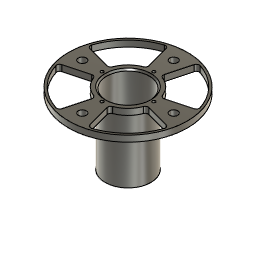
Top fan tube (Autodesk Fusion 360 design; units mm, degrees)
Autodesk Fusion 360 part; units mm, degrees
sketch "Sketch1" plane through (0, 0, 0) normal (0, 0, 1) x (1, 0, 0)
  circle A0 centre (0, 0) radius 39
  circle A1 centre (0, 0) radius 14
  circle A2 centre (0, 0) radius 17 construction
  circle A3 centre (0, 0) radius 17.5
  circle A4 centre (0, 0) radius 37.5
  line L0 (0, 0) -> (-11.368, 42.4258)
  line L1 (0, 0) -> (43.9224, 0) construction
  line L2 (0, 0) -> (10.4937, -39.163)
  line L3 (0, 0) -> (40.5446, 0) construction
  line L4 (0, 0) -> (-10.0939, -37.6711)
  line L5 (0, 0) -> (39, 0) construction
  line L6 (0, 0) -> (15.1457, 56.5247)
  line L7 (0, 0) -> (58.5186, 0) construction
  line L8 (0, 0) -> (-54.6126, 14.6334)
  line L9 (0, 0) -> (56.5391, 0) construction
  line L10 (0, 0) -> (51.9352, -13.916)
  line L11 (0, 0) -> (53.7673, 0) construction
  line L12 (0, 0) -> (-45.8179, -12.2769)
  line L13 (0, 0) -> (47.4342, 0) construction
  line L14 (0, 0) -> (50.4228, 13.5108)
  line L15 (0, 0) -> (52.2015, 0) construction
  dimension "d1" = 78
  dimension "d2" = 28
  dimension "d3" = 34
  dimension "d32" = 35
  dimension "d33" = 75
  dimension "d34" = 105
  dimension "d35" = 75
  dimension "d36" = 105
  dimension "d37" = 75
  dimension "d38" = 165
  dimension "d39" = 15
  dimension "d40" = 165
  dimension "d41" = 15
  constraint coincident A0.centre A1.centre
  constraint concentric A2 A3
  constraint horizontal L1
  constraint horizontal L3
  constraint horizontal L5
  constraint horizontal L7
  constraint horizontal L9
  constraint horizontal L11
  constraint horizontal L13
  constraint horizontal L15
  measures "d1" diameter of A0
  measures "d2" diameter of A1
  measures "d3" diameter of A2
  measures "d32" diameter of A3
  measures "d33" diameter of A4
  measures "d34" angle of L0 L1
  measures "d35" angle of L2 L3
  measures "d36" angle of L4 L5
  measures "d37" angle of L6 L7
  measures "d38" angle of L8 L9
  measures "d39" angle of L10 L11
  measures "d40" angle of L12 L13
  measures "d41" angle of L14 L15
extrude "Extrude1" add sketch "Sketch1" along normal blind 4 contours A0 A4 L10 L14 | A0 A4 L6 L14 | A0 A4 L2 L10 | A0 A4 L0 L6 | A3 A4 L6 L14 | A3 A4 L10 L14 | A0 A4 L2 L4 | A3 A4 L2 L10 | A0 A4 L0 L8 | A3 A4 L0 L6 | A1 A3 L6 L14 | A1 A3 L10 L14 | A0 A4 L4 L12 | A3 A4 L2 L4 | A1 A3 L2 L10 | A0 A4 L8 L12 | A3 A4 L0 L8 | A1 A3 L0 L6 | A3 A4 L4 L12 | A1 A3 L2 L4 | A3 A4 L8 L12 | A1 A3 L0 L8 | A1 A3 L4 L12 | A1 A3 L8 L12
sketch "Sketch2" plane through (0, 0, 4) normal (0, 0, 1) x (-1, 0, 0)
  circle A0 centre (0, 0) radius 14
  circle A1 centre (0, 0) radius 39
  line L0 (37, 0) -> (-50, 0) construction
  line L1 (0, -40) -> (0, 43.9283) construction
  circle A2 centre (17, 0) radius 1
  circle A3 centre (0, 17) radius 1
  circle A4 centre (-17, 0) radius 1
  circle A5 centre (0, -17) radius 1
  dimension "d6" = 83.9283
  dimension "d7" = 2
  dimension "d8" = 2
  dimension "d9" = 2
  dimension "d10" = 2
  constraint horizontal L0
  constraint perpendicular L0 L1
  constraint coincident L0 A2.centre
  constraint coincident L1 A3.centre
  constraint coincident L0 A4.centre
  constraint coincident L1 A5.centre
  measures "d6" distance of L1.start L1.end
  measures "d7" diameter of A2
  measures "d8" diameter of A3
  measures "d9" diameter of A4
  measures "d10" diameter of A5
extrude "Extrude2" cut sketch "Sketch2" against normal blind 5 contours A2 | A3 | A4 | A5
sketch "Sketch3" plane through (0, 0, 0) normal (0, 0, 1) x (1, 0, 0)
  circle A0 centre (0, 0) radius 30 construction
  circle A1 centre (30, -0.0028) radius 2.6
  circle A2 centre (0.0015, 30) radius 2.6
  circle A3 centre (-30, -0.0022) radius 2.6
  circle A4 centre (0.0008, -30) radius 2.6
  dimension "d13" = 60
  dimension "d14" = 5.2
  dimension "d15" = 5.2
  dimension "d16" = 5.2
  dimension "d17" = 5.2
  constraint coincident A0.centre origin
  constraint coincident A0 A1.centre
  constraint coincident A0 A2.centre
  constraint coincident A0 A3.centre
  constraint coincident A0 A4.centre
  measures "d13" diameter of A0
  measures "d14" diameter of A1
  measures "d15" diameter of A2
  measures "d16" diameter of A3
  measures "d17" diameter of A4
extrude "Extrude3" cut sketch "Sketch3" along normal blind 5
sketch "Sketch4" plane through (0, 0, 0) normal (0, 0, 1) x (1, 0, 0)
  circle A0 centre (0, 0) radius 15
  circle A1 centre (0, 0) radius 14
  dimension "d20" = 30
  dimension "d21" = 28
  constraint coincident A0.centre A1.centre
  measures "d20" diameter of A0
  measures "d21" diameter of A1
extrude "Extrude4" add sketch "Sketch4" against normal blind 43
extrude "Extrude6" cut sketch "Sketch1" along normal blind 5 contours A3 A4 L6 L14 | A3 A4 L2 L10 | A3 A4 L0 L8 | A3 A4 L4 L12
fillet "Fillet3" radius 2 15 edges at (-9.7057, -36.2222, 2) (9.7057, -36.2222, 2) (-36.2222, -9.7057, 2) (-16.9037, -4.5293, 2) (-4.5293, -16.9037, 2) (-16.9037, 4.5293, 2) (-36.2222, 9.7057, 2) (16.9037, -4.5293, 2) (36.2222, -9.7057, 2) (-9.7057, 36.2222, 2) (-4.5293, 16.9037, 2) (36.2222, 9.7057, 2) (16.9037, 4.5293, 2) (9.7057, 36.2222, 2) (4.5293, 16.9037, 2)
fillet "Fillet4" radius 2 1 edges at (4.5293, -16.9037, 2)
chamfer "Chamfer1" distance 1 angle 45 1 edges at (-13.0526, -5.0626, -43)
chamfer "Chamfer2" distance 1 angle 45 1 edges at (-13.0526, 5.0626, 4)
